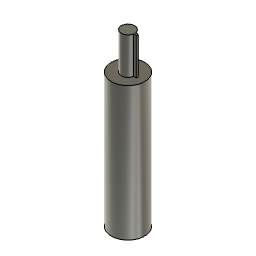
Task2 v1 (Autodesk Fusion 360 archive; units mm, degrees)
design "mtoor"
Autodesk Fusion 360 part; units mm, degrees
sketch "Sketch1" plane through (0, 0, 0) normal (0, 0, 1) x (1, 0, 0)
  circle A0 centre (0, 0) radius 50
  constraint coincident A0.centre origin
extrude "Extrude1" add sketch "Sketch1" along normal blind 400
sketch "Sketch2" plane through (0, 0, 400) normal (0, 0, 1) x (-1, 0, 0)
  circle A0 centre (0, 0) radius 50
  line L0 (-28, -3) -> (-19.7737, -3)
  line L1 (-19.7737, 3) -> (-28, 3)
  line L2 (-28, 3) -> (-28, -3)
  arc A1 (-19.7737, -3) -> (-19.7737, 3) centre (0, 0) ccw
  constraint coincident A0.centre A1.centre
  constraint horizontal L0
  constraint parallel L0 L1
extrude "Extrude2" add sketch "Sketch2" along normal blind 110 contours L0 L1 L2 A1
